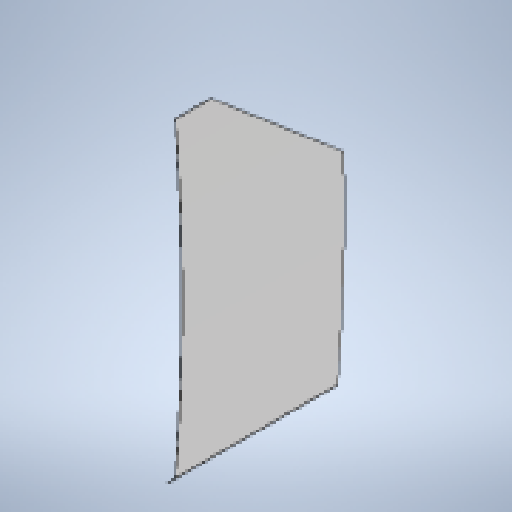
# Autodesk Inventor part: MSC 303 sheet right board withers
Saved by Autodesk Inventor 2025 (Build 290162010, 162A)
## iProperties
Created: 2024-04-18
Part Number: MSC 303 sheet right board withers
Material: AISI304
Document SubType Name: Sheet Metal
Designer: admin
Stock Number: МОО 303 лист правый борт холка
Mass: 48027.3 g
Surface Area: 40202.8 cm^2
Volume: 6003.41 cm^3
Density: 8 g/cm^3
Sheet Metal Rule: AISI304 3mm Die 32
Sheet Metal Width: 980,000 mm
Sheet Metal Length: 1948,285 mm
Sheet Metal Area: 1909318,912 mm^2
Appearance: Default
Flat Pattern Width: 98 cm
Flat Pattern Length: 194.828 cm
Flat Pattern Area: 19093.2 cm^2
Author: admin
Autodesk Inventor part; units mm, degrees
ref_plane "YZ Plane" through (0, 0, 0) normal (1, 0, 0) x (0, 1, 0)
ref_plane "XZ Plane" through (0, 0, 0) normal (0, 1, 0) x (-1, 0, 0)
ref_plane "XY Plane" through (0, 0, 0) normal (0, 0, 1) x (1, 0, 0)
sketch "Sketch1" plane through (0, 0, 0) normal (0, 0, 1) x (1, 0, 0)
  line L0 (6924.578195, -3010.685571) -> (6924.578195, -3060.685571) construction
  line L1 (0, 47) -> (0, 0) construction
  arc A0 (0.159434, 1.869277) -> (0, 1880) centre (-11009.945504, 940) ccw
  arc A1 (0, 0) -> (0.159434, 1.869277) centre (-11009.945504, 940) ccw construction
  arc A2 (-1.349222, -1.302929) -> (0.159434, 1.869277) centre (-4.822514, 2.29377) ccw
  line L2 (-1.349222, -1.302929) -> (0, 0) construction
  line L3 (-46.757087, -45.152794) -> (-1.349222, -1.302929)
  line L4 (-41.190716, -50.91694) -> (-46.757087, -45.152794) construction
  line L5 (0, 0) -> (0, 1880) construction
  line L6 (0, 0) -> (1.875639, 0) construction
  dimension "d155" = 5
  dimension "d156" = 65
  dimension "d157" = 11050
  dimension "d158" = 136
  dimension "d159" = 1880
  measures "d155" radius of A2
  measures "d156" distance of L1.end L3.start
  measures "d157" radius of A0
  measures "d158" angle of L2 L6
  measures "d159" distance of L1.end L5.end
contour flange "Contour Flange2" sketch "Sketch1" thickness 3 bend radius 5 width 980 along (0, 0, 1) mid plane no both sides no wall seen from (-24.053155, -23.227861, 0) lies toward (0.6946584, -0.7193398, 0) curves L3 A2 A0
bend "Bend2"
corner "Corner2"
sketch "Sketch2" plane through (0, 0, 0) normal (1, 0, 0) x (0, 1, 0)
  line L0 (1.614581, 980) -> (1.614581, 0)
  line L1 (1.614581, 0) -> (1880.255204, 0)
  line L2 (1880.255204, 0) -> (1880.255204, 980)
  line L3 (1.614581, 980) -> (1880.255204, 980)
  line L4 (1880.255204, 215.25) -> (1238.553761, 980)
  line L5 (1880.255204, 764.75) -> (1238.553761, 0)
  point P0 (0, 0)
  dimension "d161" = 40
  dimension "d162" = 215.25
  dimension "d164" = 215.25
  dimension "d165" = 40
  constraints: 4 end point, 4 point on line
  measures "d161" angle of L2 L4
  measures "d162" distance of L1.end L4.start
  measures "d164" distance of L2.end L5.start
  measures "d165" angle of L2 L5
extrude "Extrusion2" cut sketch "Sketch2" along normal through all both and the other way through all contours L5 L4 L2 L1 | L5 L2 L4
sketch "Sketch6" plane through (-1.349222, -1.302929, 980) normal (-0.6946584, 0.7193398, 0) x (0.7193398, 0.6946584, 0)
  line L0 (-75.255463, 38.095137) -> (-75.255463, 175.10132) construction
  line L1 (-75.255463, 175.10132) -> (-57.02188, 175.10132) construction
  line L2 (-57.02188, 175.10132) -> (-57.02188, 38.095137) construction
  line L3 (-57.02188, 38.095137) -> (-75.255463, 38.095137) construction
  point P0 (1.875639, 980)
  constraints: 2 other
feature "Mark5" [suppressed]
equation "\"d36\" = Thickness"
equation "\"GapSize\" = Thickness"
equation "\"MinimumRemnant\" = 2 * Thickness"
equation "\"BendReliefDepth\" = 0.5 * Thickness"
equation "\"BendReliefWidth\" = Thickness"
equation "\"CornerReliefSize\" = 4 * Thickness"
equation "\"d37\" = BendReliefWidth"
equation "\"d38\" = BendReliefDepth"
equation "\"d39\" = MinimumRemnant"
equation "\"d40\" = TransitionRadius"
equation "\"d42\" = BendRadius"
equation "\"d44\" = CornerReliefSize"
equation "\"d45\" = GapSize"
equation "\"d46\" = JacobiRadiusSize"
equation "\"Thickness\" = 3"
equation "\"TransitionRadius\" = 5"
equation "\"BendRadius\" = 5"
equation "\"JacobiRadiusSize\" = 5"
body "Solid3"
